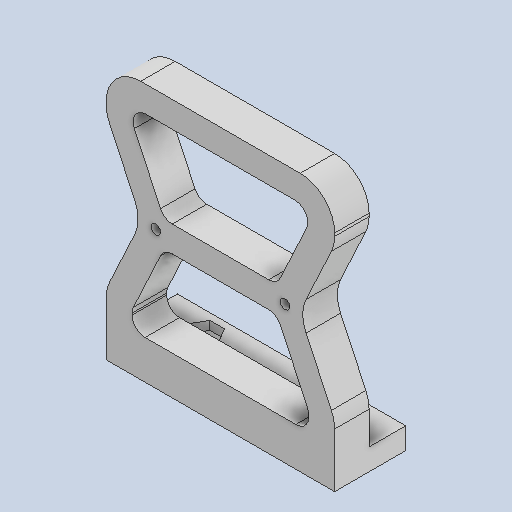
# Autodesk Inventor part: battery_mount
Saved by Autodesk Inventor 2025 (Build 290162000, 162)
## iProperties
Created: 2026-05-04
Part Number: battery_mount
Material: Generic
Document SubType Name: Modeling
Designer: Luca
Density: 1 g/cm^3
Appearance: Default
Author: Luca
Autodesk Inventor part; units mm, degrees
ref_plane "YZ Plane" through (0, 0, 0) normal (1, 0, 0) x (0, 1, 0)
ref_plane "XZ Plane" through (0, 0, 0) normal (0, 1, 0) x (-1, 0, 0)
ref_plane "XY Plane" through (0, 0, 0) normal (0, 0, 1) x (1, 0, 0)
derived "sk_reservoir.ipt"
sketch "mount" plane through (0, -70, 0) normal (0, 1, 0) x (-1, 0, 0)
  line L0 (38, -69.4029) -> (38, 38)
  line L1 (38, -55.7015) -> (40, -55.7015)
  arc A0 (40, -55.7015) -> (48, -47.7015) centre (40, -47.7015) ccw
  line L2 (48, -47.7015) -> (48, 16.2985)
  arc A1 (48, 16.2985) -> (40, 24.2985) centre (40, 16.2985) ccw
  line L3 (40, 24.2985) -> (38, 24.2985)
  line L4 (48, -15.7015) -> (38, -15.7015) construction
  line L5 (43, -55.7015) -> (43, 24.2985) construction
  line L6 (38, -55.9515) -> (40, -55.9515)
  line L7 (48.25, -47.7015) -> (48.25, 16.2985)
  line L8 (38, 24.5485) -> (40, 24.5485)
  arc A2 (48.25, 16.2985) -> (40, 24.5485) centre (40, 16.2985) ccw
  arc A3 (40, -55.9515) -> (48.25, -47.7015) centre (40, -47.7015) ccw
  line L9 (38.25, -68.9797) -> (38.25, 38.25)
  circle A4 centre (43, -15.7015) radius 1.6
  line L10 (43, -12.3015) -> (45.9445, -14.0015)
  line L11 (45.9445, -14.0015) -> (45.9445, -17.4015)
  line L12 (45.9445, -17.4015) -> (43, -19.1015)
  line L13 (43, -19.1015) -> (40.0555, -17.4015)
  line L14 (40.0555, -17.4015) -> (40.0555, -14.0015)
  line L15 (40.0555, -14.0015) -> (43, -12.3015)
  line L16 (-119, -119) -> (119, 119) construction
  arc A5 (-47.7015, 48) -> (-55.7015, 40) centre (-47.7015, 40) ccw
  line L17 (-55.7015, 38) -> (-55.7015, 40)
  line L18 (-15.7015, 48) -> (-15.7015, 38) construction
  line L19 (-47.7015, 48) -> (16.2985, 48)
  line L20 (-55.7015, 43) -> (24.2985, 43) construction
  line L21 (-69.4029, 38) -> (38, 38)
  line L22 (24.2985, 40) -> (24.2985, 38)
  arc A6 (24.2985, 40) -> (16.2985, 48) centre (16.2985, 40) ccw
  line L23 (24.5485, 38) -> (24.5485, 40)
  arc A7 (24.5485, 40) -> (16.2985, 48.25) centre (16.2985, 40) ccw
  line L24 (-14.0015, 40.0555) -> (-12.3015, 43)
  line L25 (-12.3015, 43) -> (-14.0015, 45.9445)
  line L26 (-17.4015, 40.0555) -> (-14.0015, 40.0555)
  line L27 (-14.0015, 45.9445) -> (-17.4015, 45.9445)
  circle A8 centre (-15.7015, 43) radius 1.6
  line L28 (-19.1015, 43) -> (-17.4015, 40.0555)
  line L29 (-17.4015, 45.9445) -> (-19.1015, 43)
  line L30 (-47.7015, 48.25) -> (16.2985, 48.25)
  line L31 (-68.9797, 38.25) -> (38.25, 38.25)
  arc A9 (-47.7015, 48.25) -> (-55.9515, 40) centre (-47.7015, 40) ccw
  line L32 (-55.9515, 38) -> (-55.9515, 40)
  point P0 (0, 0)
sketch "battery_mount" plane through (0, 0, 80) normal (0, 0, 1) x (1, 0, 0)
  line L0 (0, 302) -> (0, -132) construction
  line L1 (-38.25, -70) -> (68.9797, -70) construction
  line L2 (25, 0) -> (25, -57.9)
  line L3 (-25, -57.9) -> (-25, 0)
  line L4 (-25, -28.95) -> (25, -28.95) construction
  circle A0 centre (-15, -28.95) radius 1.1
  circle A1 centre (15, -28.95) radius 1.1
  line L5 (-133.1871, 0) -> (125.9572, 0)
  line L6 (-133.1871, -57.9) -> (125.9572, -57.9)
  line L7 (-24.75, -0.25) -> (24.75, -0.25)
  line L8 (24.75, -0.25) -> (24.75, -57.65)
  line L9 (24.75, -57.65) -> (-24.75, -57.65)
  line L10 (-24.75, -57.65) -> (-24.75, -0.25)
  line L11 (-26.5, -0.9) -> (26.5, -0.9)
  line L12 (-20.5, -6.9) -> (20.5, -6.9)
  line L13 (26.5, -0.9) -> (26.5, -11.3598)
  line L14 (26.5, -11.3598) -> (18.2975, -28.95)
  line L15 (18.2975, -28.95) -> (26.5, -46.5402)
  line L16 (-26.5, -0.9) -> (-26.5, -11.3598)
  line L17 (-26.5, -11.3598) -> (-18.2975, -28.95)
  line L18 (-18.2975, -28.95) -> (-26.5, -46.5402)
  line L19 (-26.5, -46.5402) -> (-26.5, -57.9)
  line L20 (26.5, -46.5402) -> (26.5, -57.9)
  line L21 (-20.5, -6.9) -> (-20.5, -10.0836)
  line L22 (-20.5, -10.0836) -> (-13.1014, -25.95)
  line L23 (-13.1014, -25.95) -> (13.1014, -25.95)
  line L24 (13.1014, -25.95) -> (20.5, -10.0836)
  line L25 (20.5, -10.0836) -> (20.5, -6.9)
  line L26 (-20.5, -51.9) -> (-20.5, -47.8164)
  line L27 (-20.5, -47.8164) -> (-13.1014, -31.95)
  line L28 (-13.1014, -31.95) -> (13.1014, -31.95)
  line L29 (13.1014, -31.95) -> (20.5, -47.8164)
  line L30 (20.5, -47.8164) -> (20.5, -51.9)
  line L31 (20.5, -51.9) -> (-20.5, -51.9)
  line L32 (-15, -28.95) -> (-24.75, -49.8589) construction
  line L33 (-18.2975, -28.95) -> (-13.1014, -31.95) construction
  line L34 (-13.1014, -31.95) -> (-13.1014, -25.95) construction
  line L35 (-20.5, -10.0836) -> (-26.5, -10.0836) construction
  line L36 (-20.5, -6.9) -> (-20.5, -0.9) construction
  line L37 (-20.5, -51.9) -> (-20.5, -57.9) construction
  line L38 (-23.5, -0.9) -> (-23.5, -57.9) construction
  line L39 (23.5, -0.9) -> (23.5, -57.9) construction
  line L40 (12.5, -28.95) -> (13.75, -26.7849)
  line L41 (13.75, -26.7849) -> (16.25, -26.7849)
  line L42 (16.25, -26.7849) -> (17.5, -28.95)
  line L43 (17.5, -28.95) -> (16.25, -31.1151)
  line L44 (16.25, -31.1151) -> (13.75, -31.1151)
  line L45 (13.75, -31.1151) -> (12.5, -28.95)
  line L46 (-17.5, -28.95) -> (-16.25, -26.7849)
  line L47 (-16.25, -26.7849) -> (-13.75, -26.7849)
  line L48 (-13.75, -26.7849) -> (-12.5, -28.95)
  line L49 (-12.5, -28.95) -> (-13.75, -31.1151)
  line L50 (-13.75, -31.1151) -> (-16.25, -31.1151)
  line L51 (-16.25, -31.1151) -> (-17.5, -28.95)
  point P0 (0, 0)
  point P1 (24.75, -42.7874)
  point P2 (24.75, -15.1126)
  point P3 (24.75, -0.9)
  point P4 (-24.75, -0.9)
  point P5 (-24.75, -15.1126)
  point P6 (-24.75, -42.7874)
sketch "battery_lid" plane through (0, -57.9, 0) normal (0, 1, 0) x (-1, 0, 0)
  arc A0 (38.25, -67.9775) -> (-67.9775, 38.25) centre (0, 0) ccw construction
  line L0 (0, -80) -> (0, 80) construction
  circle A1 centre (0, 0) radius 80
  arc A2 (-14.9031, 77.5816) -> (-20.7481, 76.2267) centre (0, 0) ccw
  arc A3 (-14.2257, 74.659) -> (-20.0707, 73.3042) centre (0, 0) ccw
  line L1 (-17.1615, 74.0393) -> (-17.8385, 76.9597) construction
  line L2 (-14.9031, 77.5816) -> (-14.2257, 74.659)
  line L3 (-20.0707, 73.3042) -> (-20.7481, 76.2267)
  arc A4 (20.2646, 72.9914) -> (-20.2646, 72.9914) centre (0, 0) ccw
  line L4 (20.2646, 72.9914) -> (21.4009, 77.0844) construction
  line L5 (-20.2646, 72.9914) -> (-21.4009, 77.0844) construction
  line L6 (-14.5278, 74.8555) -> (-15.0922, 77.2903)
  line L7 (-19.8858, 73.6136) -> (-20.4501, 76.0484)
  arc A5 (-14.5278, 74.8555) -> (-19.8858, 73.6136) centre (0, 0) ccw
  arc A6 (-15.0922, 77.2903) -> (-20.4501, 76.0484) centre (0, 0) ccw
  line L8 (25, 80) -> (-25, 80) construction
  line L9 (14.5278, 74.8555) -> (15.0922, 77.2903)
  arc A7 (20.4501, 76.0484) -> (15.0922, 77.2903) centre (0, 0) ccw
  line L10 (19.8858, 73.6136) -> (20.4501, 76.0484)
  arc A8 (19.8858, 73.6136) -> (14.5278, 74.8555) centre (0, 0) ccw
  arc A9 (20.7481, 76.2267) -> (14.9031, 77.5816) centre (0, 0) ccw
  line L11 (17.1615, 74.0393) -> (17.8385, 76.9597) construction
  arc A10 (20.0707, 73.3042) -> (14.2257, 74.659) centre (0, 0) ccw
  line L12 (20.0707, 73.3042) -> (20.7481, 76.2267)
  line L13 (14.9031, 77.5816) -> (14.2257, 74.659)
  line L14 (-27.5, 72.9914) -> (-20.2646, 72.9914)
  line L15 (20.2646, 72.9914) -> (27.5, 72.9914)
  arc A11 (-4.983, 75.5882) -> (4.983, 75.5882) centre (0, 76) ccw
  circle A12 centre (0, 76) radius 3
  arc A13 (12.7529, 78.977) -> (-12.7529, 78.977) centre (0, 71.0799) ccw
  line L16 (-29.5024, 73.2792) -> (-29.8776, 74.2114)
  line L17 (29.5024, 73.2792) -> (29.8776, 74.2114)
  line L18 (27.879, 73.9328) -> (27.5, 72.9914)
  line L19 (-27.879, 73.9328) -> (-27.5, 72.9914)
  line L20 (-28.0175, 73.6075) -> (-27.6688, 72.7414)
  line L21 (28.0175, 73.6075) -> (27.6688, 72.7414)
  line L22 (29.6409, 72.9539) -> (30.1094, 74.1176)
  line L23 (-29.6409, 72.9539) -> (-30.1094, 74.1176)
  line L24 (-20.0936, 71.7414) -> (-28.3442, 71.7414)
  line L25 (28.3442, 71.7414) -> (20.0936, 71.7414)
  arc A14 (-5.2061, 75.3225) -> (5.2061, 75.3225) centre (0, 76) ccw
  line L26 (31.0336, 73.7355) -> (30.1951, 71.6528)
  line L27 (30.1951, 71.6528) -> (28.5717, 72.3064)
  line L28 (-31.0336, 73.7355) -> (-30.1951, 71.6528)
  line L29 (-30.1951, 71.6528) -> (-28.5717, 72.3064)
  line L30 (-28.5717, 72.3064) -> (-28.3442, 71.7414)
  line L31 (28.5717, 72.3064) -> (28.3442, 71.7414)
  line L32 (-29.5024, 73.2792) -> (-27.879, 73.9328)
  line L33 (-29.6409, 72.9539) -> (-28.0175, 73.6075)
  line L34 (-29.0642, 74.5337) -> (-28.3172, 72.6783) construction
  line L35 (29.0642, 74.5337) -> (28.3172, 72.6783) construction
  line L36 (28.0175, 73.6075) -> (29.6409, 72.9539)
  line L37 (29.5024, 73.2792) -> (27.879, 73.9328)
  arc A15 (20.2305, 72.7414) -> (-20.2305, 72.7414) centre (0, 0) ccw
  line L38 (27.6688, 72.7414) -> (20.2305, 72.7414)
  line L39 (-27.6688, 72.7414) -> (-20.2305, 72.7414)
  line L40 (28.5717, 72.3064) -> (27.4912, 72.7414)
  line L41 (-28.5717, 72.3064) -> (-27.4912, 72.7414)
  arc A16 (20.0936, 71.7414) -> (-20.0936, 71.7414) centre (0, 0) ccw
  line L42 (28.5717, 72.3064) -> (28.9452, 73.234)
  line L43 (-28.5717, 72.3064) -> (-28.9452, 73.234)
  line L44 (38.25, 38.25) -> (-68.9797, 38.25) construction
  line L45 (-26.75, 38.25) -> (-26.75, 55.25)
  line L46 (-26.75, 55.25) -> (26.75, 55.25)
  line L47 (26.75, 55.25) -> (26.75, 38.25)
  line L48 (-26.75, 38.25) -> (26.75, 38.25)
  line L49 (-26.5, 38.5) -> (-26.5, 55)
  line L50 (-26.5, 55) -> (26.5, 55)
  line L51 (26.5, 55) -> (26.5, 38.5)
  line L52 (26.5, 38.5) -> (-26.5, 38.5)
  arc A17 (-6.2045, 75.2469) -> (6.2045, 75.2469) centre (0, 76) ccw
  point P0 (-25, 80)
  point P1 (25, 80)
  point P2 (-17.5, 75.4995)
  point P3 (17.5, 75.4995)
  point P4 (17.5, 75.4995)
  point P5 (-28.6907, 73.606)
  point P6 (28.6907, 73.606)
  point P7 (0, 0)
  point P8 (-26.5, 80)
  point P9 (-26.5, 80)
  point P10 (-26.5, 80)
  point P11 (26.5, 80)
  point P12 (26.5, 80)
  point P13 (26.5, 80)
extrude "Extrusion1" add sketch "battery_mount" against normal blind 8 from surface at -25 contours L11 L13 L14 L2 | L2 L14 L8 L11 | L8 L14 L15 L9 L10 L18 L17 L11 | L11 L10 L17 L3 | L3 L17 L16 L11 | L15 L20 L6 L2 | L2 L6 L3 L18 L10 L9 L8 L15 | L3 L6 L19 L18 | L40 L41 L42 L43 L44 L45 | L46 L47 L48 L49 L50 L51
extrude "Extrusion2" add sketch "battery_lid" against normal blind 3 contours L49 L50 L51 L52
extrude "Extrusion3" add sketch "battery_lid" along normal blind 2 contours L49 L50 L51 L52
extrude "Extrusion4" cut sketch "mount" along normal through all contours A8
pattern_linear "Rectangular Pattern1" count 2 spacing 31.4 along (-1, 0, 0) of "Extrusion4"
fillet "Fillet1" radius 3 12 edges at (20.5, -6.9, 51) (20.5, -10.0836, 51) (13.1014, -25.95, 51) (13.1014, -31.95, 51) (20.5, -47.8164, 51) (-20.5, -6.9, 51) (-20.5, -10.0836, 51) (-13.1014, -25.95, 51) (-20.5, -47.8164, 51) (-20.5, -51.9, 51) (-13.1014, -31.95, 51) (20.5, -51.9, 51)
fillet "Fillet2" radius 8 8 edges at (-26.5, -0.9, 51) (26.5, -0.9, 51) (26.5, -11.3598, 51) (18.2975, -28.95, 51) (26.5, -46.5402, 51) (-26.5, -11.3598, 51) (-18.2975, -28.95, 51) (-26.5, -46.5402, 51)
extrude "Extrusion5" cut sketch "mount" against normal blind 2 from surface at 14.1 contours L26 L28 L29 L27 L25 L24 | A8
pattern_linear "Rectangular Pattern2" count 2 spacing 31.4 along (-1, 0, 0) of "Extrusion5"
extrude "Extrusion6" cut sketch "battery_mount" along normal blind 1.5 from surface at -33 contours A0 | A1 | L40 L41 L42 L43 L44 L45 | L46 L47 L48 L49 L50 L51
ref_plane "Work Plane24" through (0, 0, 55) normal (0, 0, 1) x (1, 0, 0)
body "Solid1"
